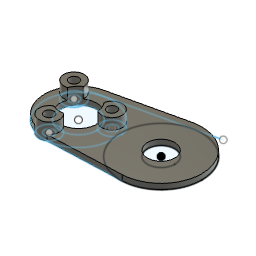
slip_ring_mount (Autodesk Fusion 360 design; units mm, degrees)
Autodesk Fusion 360 part; units mm, degrees
sketch "Sketch1" plane through (0, 0, 0) normal (0, 1, 0) x (1, 0, 0)
  circle A0 centre (0, 0) radius 15
  circle A1 centre (0, 0) radius 5
  circle A2 centre (-26.98, -3.5679) radius 12.5
  circle A3 centre (-26.98, -3.5679) radius 6.75
  line L0 (-15, 0) -> (-21.25, 0) construction
  circle A4 centre (-18.125, 0) radius 1.75
  circle A5 centre (-18.125, 0) radius 3.75
  circle A6 centre (-34.4974, 2.3169) radius 3.75
  circle A7 centre (-34.4974, 2.3169) radius 1.75
  circle A8 centre (-28.3176, -13.0204) radius 3.75
  circle A9 centre (-28.3176, -13.0204) radius 1.75
  line L1 (-26.4865, -16.0581) -> (0.5921, -14.9883)
  line L2 (-35.1738, 7.3887) -> (6.156, 16.7815)
  dimension "d8" = 30
  dimension "d9" = 10
  dimension "d10" = 25
  dimension "d11" = 13.5
  dimension "d13" = 3.5
  dimension "d14" = 2
  dimension "d16" = 360
  constraint coincident A0.centre A1.centre
  constraint concentric A2 A3
  constraint coincident A0 L0.start
  constraint coincident A2 L0.start
  constraint coincident A3 L0.end
  constraint horizontal L0
  constraint midpoint L0 A4.centre
  constraint coincident A2 L1.start
  constraint coincident A0 L1.end
  constraint tangent A0 L1
  constraint tangent A2 L1
  constraint tangent A0 L2
  constraint tangent A2 L2
  measures "d8" diameter of A0
  measures "d9" diameter of A1
  measures "d10" diameter of A2
  measures "d11" diameter of A3
  measures "d13" diameter of A4
extrude "Extrude1" add sketch "Sketch1" along normal blind 2 contours A0 A2 A5 | A0 A2 A8 L1 | A0 A2 A3 A5 A8 | A0 A2 A5 | A0 A2 A5 L2 | A2 A3 A6 A8 | A2 A3 A5 A6 picked at (-11.2572, 2.1089) picked at (-14.7409, -2.1959) makes body 1 at (-17.1331, 0, -8.9977) makes body 2 at (-33.5448, 0, 10.0531)
extrude "Extrude2" add sketch "Sketch1" along normal blind 6 contours A2 A8 L1 | A2 A8 L1 | A0 A2 A3 A5 | A0 A2 A5 | A2 A3 A8 | A0 A2 A5 | A0 A2 A5 | A2 A6 | A2 A3 A6 picked at (-14.7886, -1.2173) picked at (-14.7981, 0.3734) picked at (-15.5133, 1.9421) bodies 1 2
equation "ring_hole = 13.5 mm"
equation "ring_diam = 25 mm"
equation "screw_diam = 10 mm"
equation "depth = 2 mm"
equation "screw_od = 30 mm"
equation "insert_depth = 4 mm"
equation "insert_od = 3.5 mm"
equation "d8 = screw_od"
equation "d9 = screw_diam"
equation "d10 = ring_diam"
equation "d11 = ring_hole"
equation "m2_hole = 3 mm"
equation "d13 = insert_od"
equation "d14 = depth"
equation "d17 = depth"
equation "d19 = depth + insert_depth"
